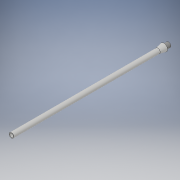
# Autodesk Inventor part: canon
Saved by Autodesk Inventor 2019 (Build 230136000, 136)
## iProperties
Created: 2019-03-19
Part Number: canon
Material: Générique
Document SubType Name: Modeling
Designer: theor
Density: 1 g/cm^3
Appearance: Par défaut
Author: theor
Autodesk Inventor part; units mm, degrees
ref_plane "YZ Plane" through (0, 0, 0) normal (1, 0, 0) x (0, 1, 0)
ref_plane "XZ Plane" through (0, 0, 0) normal (0, 1, 0) x (-1, 0, 0)
ref_plane "XY Plane" through (0, 0, 0) normal (0, 0, 1) x (1, 0, 0)
sketch "Esquisse1" plane through (0, 0, 0) normal (1, 0, 0) x (0, 1, 0)
  line L0 (0, 0) -> (0, 16.4425)
  line L1 (6, 0) -> (6, 515)
  line L2 (6, 0) -> (8, 0)
  line L3 (8, 0) -> (8, 15)
  line L4 (8, 15) -> (12, 15)
  line L5 (12, 15) -> (8, 35)
  line L6 (8, 35) -> (8, 515)
  line L7 (8, 515) -> (6, 515)
  dimension "d1" = 4
  dimension "d2" = 15
  dimension "d3" = 16
  dimension "d4" = 12
  dimension "d5" = 20
  dimension "d6" = 500
  constraints: 16 end point, 4 vertical, 3 horizontal, 1 collinear, 1 horizontal alignment
  measures "d1" distance of L3.end L4.end
  measures "d2" distance of L2.end L3.end
  measures "d3" diameter of L3 L0
  measures "d4" diameter of L1 L0
  measures "d5" vertical distance of L4.end L5.end
  measures "d6" distance between parallel lines of L7 L4
revolve "Révolution1" add sketch "Esquisse1" angle 360 about axis through (0, 0, 0) along (0, 0, 1)
thread "Filetage1" size "M16x2" class "6g" standard "ISO Metric profile" full length
